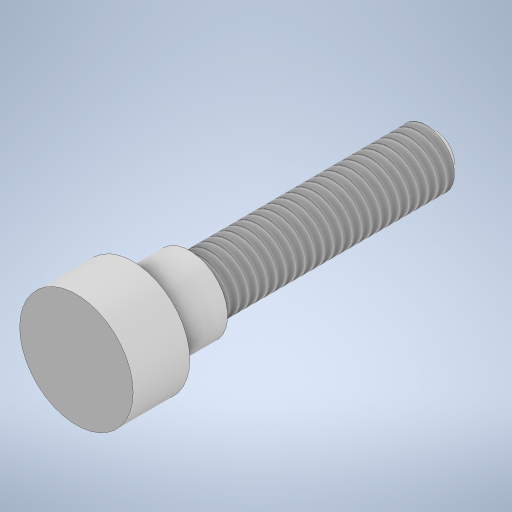
# Autodesk Inventor part: Болт М3х16
Saved by Autodesk Inventor 2023 (Build 270158000, 158)
## iProperties
Created: 2022-05-01
Part Number: Болт М3х16
Material: Типовые
Document SubType Name: Modeling
Designer: User
Density: 1 g/cm^3
Appearance: По умолчанию
Author: User
Autodesk Inventor part; units mm, degrees
ref_plane "YZ Plane" through (0, 0, 0) normal (1, 0, 0) x (0, 1, 0)
ref_plane "XZ Plane" through (0, 0, 0) normal (0, 1, 0) x (-1, 0, 0)
ref_plane "XY Plane" through (0, 0, 0) normal (0, 0, 1) x (1, 0, 0)
sketch "Эскиз1" plane through (0, 0, 0) normal (0, 1, 0) x (-1, 0, 0)
  line L0 (0, 0) -> (3, 0)
  line L1 (3, 0) -> (3, -3)
  line L2 (0, -3) -> (1.5, -3)
  line L3 (1.5, -6) -> (1.5, -19)
  line L4 (1.5, -19) -> (0, -19)
  line L5 (0, -19) -> (0, 0)
  line L6 (1.5, -3) -> (3, -3)
  line L7 (1.5, -3) -> (2, -3)
  line L8 (2, -3) -> (2, -6)
  line L9 (2, -6) -> (0, -6)
  dimension "d0" = 3
  dimension "d1" = 3
  dimension "d2" = 1.5
  dimension "d3" = 16
  dimension "d4" = 0.5
  dimension "d5" = 3
  constraints: 20 end point, 7 perpendicular, 3 point on line, 2 horizontal
  measures "d0" distance of L0.start L0.end
  measures "d1" distance of L0.end L1.end
  measures "d2" distance of L2.start L2.end
  measures "d3" distance of L2.end L3.end
  measures "d4" distance of L2.end L7.end
  measures "d5" distance of L7.end L8.end
revolve "Вращение1" add sketch "Эскиз1" angle 360 about axis through (0, 0, -19) along (0, 0, 1)
thread "Резьба1" size "M3x0.5" class "6g" standard "ISO Metric profile" full length
chamfer "Фаска1" distance 0.5 angle 45 1 edges at (1.5, 0, -19)
